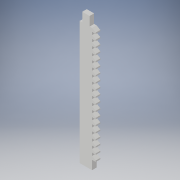
# Autodesk Inventor part: graduated_foot
Saved by Autodesk Inventor 2019.4 (Build 234330000, 330)
## iProperties
Created: 2019-12-14
Part Number: graduated_foot
Material: Generic
Document SubType Name: Modeling
Designer: fabfarm
Density: 1 g/cm^3
Appearance: Default
Author: fabfarm
Autodesk Inventor part; units mm, degrees
ref_plane "YZ Plane" through (0, 0, 0) normal (1, 0, 0) x (0, 1, 0)
ref_plane "XZ Plane" through (0, 0, 0) normal (0, 1, 0) x (-1, 0, 0)
ref_plane "XY Plane" through (0, 0, 0) normal (0, 0, 1) x (1, 0, 0)
sketch "Sketch4" plane through (0, 0, 0) normal (0, 0, 1) x (1, 0, 0)
  line L0 (0, 500) -> (50, 500)
  line L1 (50, 500) -> (50, 0)
  line L2 (50, 0) -> (0, 0)
  line L3 (0, 0) -> (0, 500)
  dimension "d31" = 50
  dimension "d32" = 500
  constraints: 8 end point, 2 parallel, 2 point on line, 1 horizontal, 1 perpendicular
  measures "d31" distance of L0.start L0.end
  measures "d32" distance of L2.end L0.start
extrude "Extrusion1" add sketch "Sketch4" along normal blind 18.55
sketch "Sketch5" plane through (0, 0, 18.55) normal (0, 0, 1) x (1, 0, 0)
  line L0 (50, 500) -> (0, 500) projected
  line L1 (10, 500) -> (40, 500)
  line L2 (40, 500) -> (40, 537.1)
  line L3 (40, 537.1) -> (10, 537.1)
  line L4 (10, 537.1) -> (10, 500)
  line L5 (0, 500) -> (0, 0) projected
  line L6 (50, 0) -> (50, 500) projected
  dimension "d46" = 10
  dimension "d47" = 10
  dimension "d48" = 37.1
  constraints: 8 end point, 2 parallel, 1 horizontal, 1 perpendicular, 1 point on line
  measures "d46" distance between parallel lines of L5 L4
  measures "d47" distance between parallel lines of L6 L2
  measures "d48" distance of L3.end L1.start
extrude "Extrusion2" add sketch "Sketch5" against normal blind 18.55
sketch "Sketch6" plane through (0, 0, 18.55) normal (0, 0, 1) x (1, 0, 0)
  line L0 (50, 500) -> (65, 491.3397)
  line L1 (65, 491.3397) -> (65, 486.3397)
  line L2 (65, 486.3397) -> (50, 486.3397)
  line L3 (50, 500) -> (40, 500) projected
  line L4 (40, 500) -> (50, 500) projected
  line L5 (50, 500) -> (50, 486.3397)
  line L6 (50, 0) -> (50, 500) projected
  line L7 (50, 475) -> (65, 466.3397)
  line L8 (65, 466.3397) -> (65, 461.3397)
  line L9 (65, 461.3397) -> (50, 461.3397)
  line L10 (50, 475) -> (50, 461.3397)
  line L11 (50, 450) -> (65, 441.3397)
  line L12 (65, 441.3397) -> (65, 436.3397)
  line L13 (65, 436.3397) -> (50, 436.3397)
  line L14 (50, 450) -> (50, 436.3397)
  line L15 (50, 425) -> (65, 416.3397)
  line L16 (65, 416.3397) -> (65, 411.3397)
  line L17 (65, 411.3397) -> (50, 411.3397)
  line L18 (50, 425) -> (50, 411.3397)
  line L19 (50, 400) -> (65, 391.3397)
  line L20 (65, 391.3397) -> (65, 386.3397)
  line L21 (65, 386.3397) -> (50, 386.3397)
  line L22 (50, 400) -> (50, 386.3397)
  line L23 (50, 375) -> (65, 366.3397)
  line L24 (65, 366.3397) -> (65, 361.3397)
  line L25 (65, 361.3397) -> (50, 361.3397)
  line L26 (50, 375) -> (50, 361.3397)
  line L27 (50, 350) -> (65, 341.3397)
  line L28 (65, 341.3397) -> (65, 336.3397)
  line L29 (65, 336.3397) -> (50, 336.3397)
  line L30 (50, 350) -> (50, 336.3397)
  line L31 (50, 325) -> (65, 316.3397)
  line L32 (65, 316.3397) -> (65, 311.3397)
  line L33 (65, 311.3397) -> (50, 311.3397)
  line L34 (50, 325) -> (50, 311.3397)
  line L35 (50, 300) -> (65, 291.3397)
  line L36 (65, 291.3397) -> (65, 286.3397)
  line L37 (65, 286.3397) -> (50, 286.3397)
  line L38 (50, 300) -> (50, 286.3397)
  line L39 (50, 275) -> (65, 266.3397)
  line L40 (65, 266.3397) -> (65, 261.3397)
  line L41 (65, 261.3397) -> (50, 261.3397)
  line L42 (50, 275) -> (50, 261.3397)
  line L43 (50, 250) -> (65, 241.3397)
  line L44 (65, 241.3397) -> (65, 236.3397)
  line L45 (65, 236.3397) -> (50, 236.3397)
  line L46 (50, 250) -> (50, 236.3397)
  line L47 (50, 225) -> (65, 216.3397)
  line L48 (65, 216.3397) -> (65, 211.3397)
  line L49 (65, 211.3397) -> (50, 211.3397)
  line L50 (50, 225) -> (50, 211.3397)
  line L51 (50, 200) -> (65, 191.3397)
  line L52 (65, 191.3397) -> (65, 186.3397)
  line L53 (65, 186.3397) -> (50, 186.3397)
  line L54 (50, 200) -> (50, 186.3397)
  line L55 (50, 175) -> (65, 166.3397)
  line L56 (65, 166.3397) -> (65, 161.3397)
  line L57 (65, 161.3397) -> (50, 161.3397)
  line L58 (50, 175) -> (50, 161.3397)
  line L59 (50, 150) -> (65, 141.3397)
  line L60 (65, 141.3397) -> (65, 136.3397)
  line L61 (65, 136.3397) -> (50, 136.3397)
  line L62 (50, 150) -> (50, 136.3397)
  line L63 (50, 125) -> (65, 116.3397)
  line L64 (65, 116.3397) -> (65, 111.3397)
  line L65 (65, 111.3397) -> (50, 111.3397)
  line L66 (50, 125) -> (50, 111.3397)
  line L67 (50, 100) -> (65, 91.3397)
  line L68 (65, 91.3397) -> (65, 86.3397)
  line L69 (65, 86.3397) -> (50, 86.3397)
  line L70 (50, 100) -> (50, 86.3397)
  line L71 (50, 75) -> (65, 66.3397)
  line L72 (65, 66.3397) -> (65, 61.3397)
  line L73 (65, 61.3397) -> (50, 61.3397)
  line L74 (50, 75) -> (50, 61.3397)
  line L75 (50, 50) -> (65, 41.3397)
  line L76 (65, 41.3397) -> (65, 36.3397)
  line L77 (65, 36.3397) -> (50, 36.3397)
  line L78 (50, 50) -> (50, 36.3397)
  line L79 (50, 25) -> (65, 16.3397)
  line L80 (65, 16.3397) -> (65, 11.3397)
  line L81 (65, 11.3397) -> (50, 11.3397)
  line L82 (50, 25) -> (50, 11.3397)
  point P0 (0, 0)
  point P1 (40, 475)
  point P2 (40, 450)
  point P3 (40, 425)
  point P4 (40, 400)
  point P5 (40, 375)
  point P6 (40, 350)
  point P7 (40, 325)
  point P8 (40, 300)
  point P9 (40, 275)
  point P10 (40, 250)
  point P11 (40, 225)
  point P12 (40, 200)
  point P13 (40, 175)
  point P14 (40, 150)
  point P15 (40, 125)
  point P16 (40, 100)
  point P17 (40, 75)
  point P18 (40, 50)
  point P19 (40, 25)
  dimension "d49" = 15
  dimension "d50" = 30
  dimension "d51" = 5
  dimension "d54" = 25
  constraints: 160 end point, 1 collinear, 1 horizontal, 1 perpendicular, 1 vertical, 171 other
  measures "d49" distance of L1.end L2.end
  measures "d50" angle of L3 L0
  measures "d51" distance of L0.end L1.end
  measures "d54" distance of L0.start L7.start
extrude "Extrusion3" add sketch "Sketch6" against normal blind 18.55 contours L75 L76 L77 L6 | L71 L72 L73 L6 | L67 L68 L69 L6 | L63 L64 L65 L6 | L59 L60 L61 L6 | L55 L56 L57 L6 | L51 L52 L53 L6 | L47 L48 L49 L6 | L43 L44 L45 L6 | L39 L40 L41 L6 | L35 L36 L37 L6 | L31 L32 L33 L6 | L27 L28 L29 L6 | L23 L24 L25 L6 | L19 L20 L21 L6 | L15 L16 L17 L6 | L11 L12 L13 L6 | L7 L8 L9 L6 | L0 L1 L2 L5
body "Solid1"
